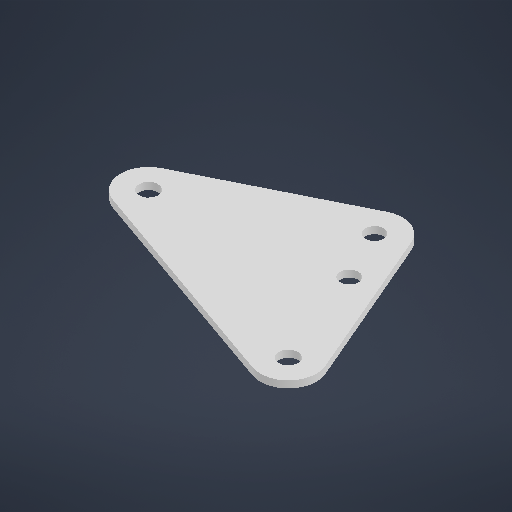
# Autodesk Inventor part: newstackpoly
Saved by Autodesk Inventor 2025.2 (Build 292293000, 293)
## iProperties
Created: 2025-04-03
Part Number: newstackpoly
Material: Generic
Document SubType Name: Modeling
Designer: Jahan
Density: 1 g/cm^3
Appearance: Default
Author: Jahan
Autodesk Inventor part; units mm, degrees
ref_plane "YZ Plane" through (0, 0, 0) normal (1, 0, 0) x (0, 1, 0)
ref_plane "XZ Plane" through (0, 0, 0) normal (0, 1, 0) x (-1, 0, 0)
ref_plane "XY Plane" through (0, 0, 0) normal (0, 0, 1) x (1, 0, 0)
sketch "Sketch1" plane through (0, 0, 0) normal (0, 1, 0) x (-1, 0, 0)
  circle A0 centre (-25.0009, 13.9426) radius 2.1844
  circle A1 centre (-10.4764, -20.0504) radius 2.0828
  circle A2 centre (-16.132, -8.6792) radius 2.0828
  circle A3 centre (0.8946, -14.3946) radius 2.0828
  circle A4 centre (12.266, -8.7393) radius 2.1844
  circle A5 centre (23.6373, -3.084) radius 2.1844
  circle A6 centre (-25.0009, 13.9426) radius 6.35
  circle A7 centre (-10.4764, -20.0504) radius 6.35
  circle A8 centre (23.6373, -3.084) radius 6.35
  line L0 (-30.8402, 11.4476) -> (-16.3157, -22.5454)
  line L1 (-22.9029, 19.936) -> (25.7354, 2.9094)
  line L2 (26.4651, -8.7697) -> (-7.6487, -25.736)
  point P0 (0, 0)
  dimension "d0" = 12.7
  dimension "d1" = 12.7
  dimension "d3" = 12.7
  constraints: 9 centre point, 6 end point, 6 point on circle, 6 tangent, 3 coincident
  measures "d0" diameter of A6
  measures "d1" diameter of A7
  measures "d3" diameter of A8
extrude "Extrusion1" add sketch "Sketch1" along normal blind 1.5875 contours A3 | A4 | A6 | A6 L1 A8 L2 A7 L0 | A8 | A7
body "Solid1"
